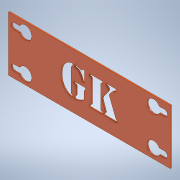
# Autodesk Inventor part: Head_GK_cloth
Saved by Autodesk Inventor 2020.4 (Build 244396000, 396)
## iProperties
Created: 2022-06-21
Part Number: Head_GK_cloth
Material: 一般
Document SubType Name: Modeling
Designer: Masato Kubotera
Density: 1 g/cm^3
Appearance: 滑らか - 淡いオレンジ
Author: Masato Kubotera
Autodesk Inventor part; units mm, degrees
ref_plane "YZ Plane" through (0, 0, 0) normal (1, 0, 0) x (0, 1, 0)
ref_plane "XZ Plane" through (0, 0, 0) normal (0, 1, 0) x (-1, 0, 0)
ref_plane "XY Plane" through (0, 0, 0) normal (0, 0, 1) x (1, 0, 0)
sketch "スケッチ1" plane through (0, 0, 0) normal (1, 0, 0) x (0, 1, 0)
  line L0 (-56.1, 19) -> (56.1, 19)
  line L1 (56.1, 19) -> (56.1, -19)
  line L2 (56.1, -19) -> (-56.1, -19)
  line L3 (-56.1, -19) -> (-56.1, 19)
  line L4 (-56.1, 19) -> (56.1, -19) construction
  line L5 (56.1, 19) -> (-56.1, -19) construction
  arc A0 (-48.4799, 10.4) -> (-48.4799, 14.6) centre (-44.5, 12.5) ccw
  line L6 (-52, 10.4) -> (-48.4799, 10.4)
  line L7 (-52, 14.6) -> (-48.4799, 14.6)
  arc A1 (-52, 14.6) -> (-52, 10.4) centre (-52, 12.5) ccw
  line L8 (-52, 12.5) -> (-44.5, 12.5) construction
  line L9 (-56.1, 0) -> (56.1, 0) construction
  line L10 (-52, 19) -> (-52, -19) construction
  line L11 (-56.1, -19) -> (56.1, 19) construction
  line L12 (-52, -14.6) -> (-48.4799, -14.6)
  arc A2 (-52, -10.4) -> (-52, -14.6) centre (-52, -12.5) ccw
  line L13 (-52, -10.4) -> (-48.4799, -10.4)
  arc A3 (-48.4799, -14.6) -> (-48.4799, -10.4) centre (-44.5, -12.5) ccw
  line L14 (-52, -12.5) -> (-44.5, -12.5) construction
  line L15 (-52, -19) -> (-52, 19) construction
  line L16 (0, 19) -> (0, -19) construction
  line L17 (56.1, 19) -> (-56.1, -19) construction
  line L18 (-56.1, 19) -> (56.1, -19) construction
  line L19 (52, 14.6) -> (48.4799, 14.6)
  arc A4 (52, 10.4) -> (52, 14.6) centre (52, 12.5) ccw
  line L20 (52, 10.4) -> (48.4799, 10.4)
  arc A5 (48.4799, 14.6) -> (48.4799, 10.4) centre (44.5, 12.5) ccw
  line L21 (52, 12.5) -> (44.5, 12.5) construction
  line L22 (56.1, 0) -> (-56.1, 0) construction
  line L23 (52, 19) -> (52, -19) construction
  arc A6 (52, -14.6) -> (52, -10.4) centre (52, -12.5) ccw
  line L24 (52, -14.6) -> (48.4799, -14.6)
  line L25 (52, -10.4) -> (48.4799, -10.4)
  line L26 (52, -12.5) -> (44.5, -12.5) construction
  arc A7 (48.4799, -10.4) -> (48.4799, -14.6) centre (44.5, -12.5) ccw
  line L27 (52, -19) -> (52, 19) construction
  line L28 (56.1, -19) -> (-56.1, 19) construction
  line L29 (-9.8507, 5.0432) -> (9.8507, 5.0432) construction
  line L30 (9.8507, 5.0432) -> (9.8507, -5.0432) construction
  line L31 (9.8507, -5.0432) -> (-9.8507, -5.0432) construction
  line L32 (-9.8507, -5.0432) -> (-9.8507, 5.0432) construction
  line L33 (-9.8507, 5.0432) -> (9.8507, -5.0432) construction
  line L34 (9.8507, 5.0432) -> (-9.8507, -5.0432) construction
  line L35 (-11.4757, 10.3993) -> (-11.4757, 8.7674)
  spline S0 degree 2 poles (-11.4757, 8.7674) (-12.7604, 8.4549) (-12.7604, 6.7187) knots 0 0 0 1 1 1
  line L36 (-12.7604, 6.7187) -> (-12.7604, -6.9271)
  spline S1 degree 2 poles (-12.7604, -6.9271) (-12.7604, -7.7083) (-12.5347, -8.1424) knots 0 0 0 1 1 1
  spline S2 degree 2 poles (-12.5347, -8.1424) (-12.3437, -8.4896) (-11.7361, -8.7326) knots 0 0 0 1 1 1
  line L37 (-11.7361, -8.7326) -> (-11.7361, -10.3993)
  spline S3 degree 2 poles (-11.7361, -10.3993) (-12.2049, -10.3993) (-12.9861, -10.2431) (-13.6285, -10.0347) knots 0 0 0 1 2 2 2
  spline S4 degree 2 poles (-13.6285, -10.0347) (-15.1562, -9.4965) (-17.6562, -7.3264) (-18.4549, -5.816) knots 0 0 0 1 2 2 2
  spline S5 degree 2 poles (-18.4549, -5.816) (-19.7049, -3.4722) (-19.7049, -0.2431) knots 0 0 0 1 1 1
  spline S6 degree 2 poles (-19.7049, -0.2431) (-19.7049, 2.8819) (-17.4826, 7.7083) (-15.3993, 9.0972) knots 0 0 0 1 2 2 2
  spline S7 degree 2 poles (-15.3993, 9.0972) (-14.2014, 9.8958) (-12.8299, 10.2431) knots 0 0 0 1 1 1
  spline S8 degree 2 poles (-12.8299, 10.2431) (-12.2569, 10.3993) (-11.4757, 10.3993) knots 0 0 0 1 1 1
  spline S9 degree 2 poles (-3.6632, -7.5521) (-4.2535, -8.1424) (-6.1979, -9.3576) (-7.066, -9.7049) knots 0 0 0 1 2 2 2
  spline S10 degree 2 poles (-7.066, -9.7049) (-7.8472, -10.0174) (-9.7743, -10.3993) (-10.5035, -10.3993) knots 0 0 0 1 2 2 2
  line L38 (-10.5035, -10.3993) -> (-10.5035, -8.7326)
  spline S11 degree 2 poles (-10.5035, -8.7326) (-10.0694, -8.6458) (-9.6528, -8.3507) (-9.4965, -8.0729) knots 0 0 0 1 2 2 2
  spline S12 degree 2 poles (-9.4965, -8.0729) (-9.2535, -7.6215) (-9.2535, -6.9271) knots 0 0 0 1 1 1
  line L39 (-9.2535, -6.9271) -> (-9.2535, -2.6389)
  spline S13 degree 2 poles (-9.2535, -2.6389) (-9.2535, -2.066) (-9.4792, -1.8229) knots 0 0 0 1 1 1
  spline S14 degree 2 poles (-9.4792, -1.8229) (-9.5833, -1.684) (-9.7743, -1.5972) (-10.3472, -1.4757) knots 0 0 0 1 2 2 2
  spline S15 degree 2 poles (-10.3472, -1.4757) (-11.059, -1.3021) (-11.059, -0.6597) knots 0 0 0 1 1 1
  spline S16 degree 2 poles (-11.059, -0.6597) (-11.059, -0.2778) (-10.3993, 0.1389) (-9.7569, 0.1389) knots 0 0 0 1 2 2 2
  line L40 (-9.7569, 0.1389) -> (-9.2708, 0.1389)
  line L41 (-9.2708, 0.1389) -> (-3.9062, 0.1389)
  spline S17 degree 2 poles (-3.9062, 0.1389) (-3.2465, 0.1389) (-2.7083, -0.2257) (-2.7083, -0.6771) knots 0 0 0 1 2 2 2
  spline S18 degree 2 poles (-2.7083, -0.6771) (-2.7083, -0.9549) (-2.934, -1.3194) (-3.2292, -1.5278) knots 0 0 0 1 2 2 2
  spline S19 degree 2 poles (-3.2292, -1.5278) (-3.5243, -1.7361) (-3.6632, -2.0833) (-3.6632, -2.5521) knots 0 0 0 1 2 2 2
  line L42 (-3.6632, -2.5521) -> (-3.6632, -7.5521)
  line L43 (-10.2778, 8.8021) -> (-10.2778, 10.3819)
  spline S20 degree 2 poles (-10.2778, 10.3819) (-7.8993, 10.1562) (-6.3542, 9.4965) knots 0 0 0 1 1 1
  spline S21 degree 2 poles (-6.3542, 9.4965) (-5.9028, 9.2882) (-5.6597, 9.2882) knots 0 0 0 1 1 1
  spline S22 degree 2 poles (-5.6597, 9.2882) (-5.4167, 9.2882) (-5.1736, 9.5139) (-4.7917, 10.0347) knots 0 0 0 1 2 2 2
  spline S23 degree 2 poles (-4.7917, 10.0347) (-4.5312, 10.3993) (-4.1319, 10.3993) knots 0 0 0 1 1 1
  spline S24 degree 2 poles (-4.1319, 10.3993) (-3.7153, 10.3993) (-3.3854, 9.9479) (-3.3854, 9.4097) knots 0 0 0 1 2 2 2
  line L44 (-3.3854, 9.4097) -> (-3.3854, 3.7153)
  spline S25 degree 2 poles (-3.3854, 3.7153) (-3.3854, 2.5868) (-4.2014, 2.5868) knots 0 0 0 1 1 1
  spline S26 degree 2 poles (-4.2014, 2.5868) (-4.6181, 2.5868) (-5.0174, 3.0208) (-5.191, 3.6806) knots 0 0 0 1 2 2 2
  spline S27 degree 2 poles (-5.191, 3.6806) (-5.3993, 4.4965) (-6.5451, 6.684) (-7.066, 7.309) knots 0 0 0 1 2 2 2
  spline S28 degree 2 poles (-7.066, 7.309) (-7.6736, 8.0556) (-9.1667, 8.7326) (-10.2778, 8.8021) knots 0 0 0 1 2 2 2
  line L45 (7.8299, -10) -> (1.2847, -10)
  line L46 (1.2847, -10) -> (0.9028, -10)
  spline S29 degree 2 poles (0.9028, -10) (0.3819, -10) (-0.191, -9.6007) (-0.191, -9.2361) knots 0 0 0 1 2 2 2
  spline S30 degree 2 poles (-0.191, -9.2361) (-0.191, -8.6458) (0.3993, -8.4549) knots 0 0 0 1 1 1
  spline S31 degree 2 poles (0.3993, -8.4549) (0.8854, -8.2813) (1.0417, -8.2118) (1.1285, -8.0729) knots 0 0 0 1 2 2 2
  spline S32 degree 2 poles (1.1285, -8.0729) (1.3021, -7.8472) (1.3021, -7.3264) knots 0 0 0 1 1 1
  line L47 (1.3021, -7.3264) -> (1.3021, 7.3264)
  spline S33 degree 2 poles (1.3021, 7.3264) (1.3021, 7.8472) (1.1285, 8.0729) knots 0 0 0 1 1 1
  spline S34 degree 2 poles (1.1285, 8.0729) (1.0417, 8.2118) (0.8854, 8.2812) (0.3993, 8.4375) knots 0 0 0 1 2 2 2
  spline S35 degree 2 poles (0.3993, 8.4375) (-0.191, 8.6285) (-0.191, 9.2361) knots 0 0 0 1 1 1
  spline S36 degree 2 poles (-0.191, 9.2361) (-0.191, 9.6007) (0.3819, 10) (0.9028, 10) knots 0 0 0 1 2 2 2
  line L48 (0.9028, 10) -> (1.2847, 10)
  line L49 (1.2847, 10) -> (7.8299, 10)
  line L50 (7.8299, 10) -> (8.2118, 10)
  spline S37 degree 2 poles (8.2118, 10) (8.7326, 10) (9.3056, 9.6007) (9.3056, 9.2361) knots 0 0 0 1 2 2 2
  spline S38 degree 2 poles (9.3056, 9.2361) (9.3056, 8.6285) (8.7153, 8.4375) knots 0 0 0 1 1 1
  spline S39 degree 2 poles (8.7153, 8.4375) (8.2292, 8.2812) (8.0729, 8.2118) (7.9861, 8.0729) knots 0 0 0 1 2 2 2
  spline S40 degree 2 poles (7.9861, 8.0729) (7.8125, 7.8472) (7.8125, 7.3264) knots 0 0 0 1 1 1
  line L51 (7.8125, 7.3264) -> (7.8125, -7.3264)
  spline S41 degree 2 poles (7.8125, -7.3264) (7.8125, -8.1597) (8.2465, -8.2986) knots 0 0 0 1 1 1
  line L52 (8.2465, -8.2986) -> (8.6979, -8.4549)
  spline S42 degree 2 poles (8.6979, -8.4549) (9.2535, -8.6285) (9.2535, -9.2361) knots 0 0 0 1 1 1
  spline S43 degree 2 poles (9.2535, -9.2361) (9.2535, -10) (8.2118, -10) knots 0 0 0 1 1 1
  line L53 (8.2118, -10) -> (7.8299, -10)
  line L54 (13.6285, 4.184) -> (18.0556, -7.3785)
  spline S44 degree 2 poles (18.0556, -7.3785) (18.2292, -7.8472) (18.6111, -8.3333) (18.9062, -8.4549) knots 0 0 0 1 2 2 2
  spline S45 degree 2 poles (18.9062, -8.4549) (19.2188, -8.6111) (19.3056, -8.6806) knots 0 0 0 1 1 1
  spline S46 degree 2 poles (19.3056, -8.6806) (19.5139, -8.8889) (19.5139, -9.2188) knots 0 0 0 1 1 1
  spline S47 degree 2 poles (19.5139, -9.2188) (19.5139, -10) (18.4028, -10) knots 0 0 0 1 1 1
  line L55 (18.4028, -10) -> (11.0417, -10)
  spline S48 degree 2 poles (11.0417, -10) (10.5208, -10) (9.9479, -9.566) (9.9479, -9.1493) knots 0 0 0 1 2 2 2
  spline S49 degree 2 poles (9.9479, -9.1493) (9.9479, -8.6806) (10.4861, -8.4201) knots 0 0 0 1 1 1
  spline S50 degree 2 poles (10.4861, -8.4201) (10.8333, -8.2639) (11.059, -8.0382) (11.0764, -7.8472) knots 0 0 0 1 2 2 2
  spline S51 degree 2 poles (11.0764, -7.8472) (11.0764, -7.7431) (10.9549, -7.3785) knots 0 0 0 1 1 1
  line L56 (10.9549, -7.3785) -> (9.0799, -1.7882)
  spline S52 degree 2 poles (9.0799, -1.7882) (8.8194, -1.0069) (8.8194, -0.4688) knots 0 0 0 1 1 1
  spline S53 degree 2 poles (8.8194, -0.4688) (8.8194, 0.0521) (9.2361, 0.6597) knots 0 0 0 1 1 1
  line L57 (9.2361, 0.6597) -> (12.7431, 5.5903)
  spline S54 degree 2 poles (12.7431, 5.5903) (13.2465, 6.2847) (13.2465, 7.0312) knots 0 0 0 1 1 1
  spline S55 degree 2 poles (13.2465, 7.0312) (13.2465, 7.4306) (12.8125, 8.1424) (12.4306, 8.2812) knots 0 0 0 1 2 2 2
  line L58 (12.4306, 8.2812) -> (11.9097, 8.5069)
  spline S56 degree 2 poles (11.9097, 8.5069) (11.4063, 8.7153) (11.4063, 9.2014) knots 0 0 0 1 1 1
  spline S57 degree 2 poles (11.4063, 9.2014) (11.4063, 9.5833) (11.7188, 9.8437) knots 0 0 0 1 1 1
  spline S58 degree 2 poles (11.7188, 9.8437) (11.9271, 10) (12.3958, 10) knots 0 0 0 1 1 1
  line L59 (12.3958, 10) -> (17.6042, 10)
  spline S59 degree 2 poles (17.6042, 10) (18.125, 10) (18.6979, 9.5486) (18.6979, 9.1319) knots 0 0 0 1 2 2 2
  spline S60 degree 2 poles (18.6979, 9.1319) (18.6979, 8.5243) (18.0208, 8.2465) knots 0 0 0 1 1 1
  line L60 (18.0208, 8.2465) -> (17.2396, 7.9514)
  spline S61 degree 2 poles (17.2396, 7.9514) (16.7535, 7.7778) (16.0069, 7.1528) knots 0 0 0 1 1 1
  spline S62 degree 2 poles (16.0069, 7.1528) (15.4514, 6.684) (14.6354, 5.5903) knots 0 0 0 1 1 1
  line L61 (14.6354, 5.5903) -> (13.6285, 4.184)
  line L62 (-11.4757, 10.3993) -> (-11.4757, 8.7674)
  spline S63 degree 2 poles (-11.4757, 8.7674) (-12.7604, 8.4549) (-12.7604, 6.7187) knots 0 0 0 1 1 1
  line L63 (-12.7604, 6.7187) -> (-12.7604, -6.9271)
  spline S64 degree 2 poles (-12.7604, -6.9271) (-12.7604, -7.7083) (-12.5347, -8.1424) knots 0 0 0 1 1 1
  spline S65 degree 2 poles (-12.5347, -8.1424) (-12.3437, -8.4896) (-11.7361, -8.7326) knots 0 0 0 1 1 1
  line L64 (-11.7361, -8.7326) -> (-11.7361, -10.3993)
  spline S66 degree 2 poles (-11.7361, -10.3993) (-12.2049, -10.3993) (-12.9861, -10.2431) (-13.6285, -10.0347) knots 0 0 0 1 2 2 2
  spline S67 degree 2 poles (-13.6285, -10.0347) (-15.1562, -9.4965) (-17.6562, -7.3264) (-18.4549, -5.816) knots 0 0 0 1 2 2 2
  spline S68 degree 2 poles (-18.4549, -5.816) (-19.7049, -3.4722) (-19.7049, -0.2431) knots 0 0 0 1 1 1
  spline S69 degree 2 poles (-19.7049, -0.2431) (-19.7049, 2.8819) (-17.4826, 7.7083) (-15.3993, 9.0972) knots 0 0 0 1 2 2 2
  spline S70 degree 2 poles (-15.3993, 9.0972) (-14.2014, 9.8958) (-12.8299, 10.2431) knots 0 0 0 1 1 1
  spline S71 degree 2 poles (-12.8299, 10.2431) (-12.2569, 10.3993) (-11.4757, 10.3993) knots 0 0 0 1 1 1
  spline S72 degree 2 poles (-3.6632, -7.5521) (-4.2535, -8.1424) (-6.1979, -9.3576) (-7.066, -9.7049) knots 0 0 0 1 2 2 2
  spline S73 degree 2 poles (-7.066, -9.7049) (-7.8472, -10.0174) (-9.7743, -10.3993) (-10.5035, -10.3993) knots 0 0 0 1 2 2 2
  line L65 (-10.5035, -10.3993) -> (-10.5035, -8.7326)
  spline S74 degree 2 poles (-10.5035, -8.7326) (-10.0694, -8.6458) (-9.6528, -8.3507) (-9.4965, -8.0729) knots 0 0 0 1 2 2 2
  spline S75 degree 2 poles (-9.4965, -8.0729) (-9.2535, -7.6215) (-9.2535, -6.9271) knots 0 0 0 1 1 1
  line L66 (-9.2535, -6.9271) -> (-9.2535, -2.6389)
  spline S76 degree 2 poles (-9.2535, -2.6389) (-9.2535, -2.066) (-9.4792, -1.8229) knots 0 0 0 1 1 1
  spline S77 degree 2 poles (-9.4792, -1.8229) (-9.5833, -1.684) (-9.7743, -1.5972) (-10.3472, -1.4757) knots 0 0 0 1 2 2 2
  spline S78 degree 2 poles (-10.3472, -1.4757) (-11.059, -1.3021) (-11.059, -0.6597) knots 0 0 0 1 1 1
  spline S79 degree 2 poles (-11.059, -0.6597) (-11.059, -0.2778) (-10.3993, 0.1389) (-9.7569, 0.1389) knots 0 0 0 1 2 2 2
  line L67 (-9.7569, 0.1389) -> (-9.2708, 0.1389)
  line L68 (-9.2708, 0.1389) -> (-3.9062, 0.1389)
  spline S80 degree 2 poles (-3.9062, 0.1389) (-3.2465, 0.1389) (-2.7083, -0.2257) (-2.7083, -0.6771) knots 0 0 0 1 2 2 2
  spline S81 degree 2 poles (-2.7083, -0.6771) (-2.7083, -0.9549) (-2.934, -1.3194) (-3.2292, -1.5278) knots 0 0 0 1 2 2 2
  spline S82 degree 2 poles (-3.2292, -1.5278) (-3.5243, -1.7361) (-3.6632, -2.0833) (-3.6632, -2.5521) knots 0 0 0 1 2 2 2
  line L69 (-3.6632, -2.5521) -> (-3.6632, -7.5521)
  line L70 (-10.2778, 8.8021) -> (-10.2778, 10.3819)
  spline S83 degree 2 poles (-10.2778, 10.3819) (-7.8993, 10.1562) (-6.3542, 9.4965) knots 0 0 0 1 1 1
  spline S84 degree 2 poles (-6.3542, 9.4965) (-5.9028, 9.2882) (-5.6597, 9.2882) knots 0 0 0 1 1 1
  spline S85 degree 2 poles (-5.6597, 9.2882) (-5.4167, 9.2882) (-5.1736, 9.5139) (-4.7917, 10.0347) knots 0 0 0 1 2 2 2
  spline S86 degree 2 poles (-4.7917, 10.0347) (-4.5312, 10.3993) (-4.1319, 10.3993) knots 0 0 0 1 1 1
  spline S87 degree 2 poles (-4.1319, 10.3993) (-3.7153, 10.3993) (-3.3854, 9.9479) (-3.3854, 9.4097) knots 0 0 0 1 2 2 2
  line L71 (-3.3854, 9.4097) -> (-3.3854, 3.7153)
  spline S88 degree 2 poles (-3.3854, 3.7153) (-3.3854, 2.5868) (-4.2014, 2.5868) knots 0 0 0 1 1 1
  spline S89 degree 2 poles (-4.2014, 2.5868) (-4.6181, 2.5868) (-5.0174, 3.0208) (-5.191, 3.6806) knots 0 0 0 1 2 2 2
  spline S90 degree 2 poles (-5.191, 3.6806) (-5.3993, 4.4965) (-6.5451, 6.684) (-7.066, 7.309) knots 0 0 0 1 2 2 2
  spline S91 degree 2 poles (-7.066, 7.309) (-7.6736, 8.0556) (-9.1667, 8.7326) (-10.2778, 8.8021) knots 0 0 0 1 2 2 2
  line L72 (7.8299, -10) -> (1.2847, -10)
  line L73 (1.2847, -10) -> (0.9028, -10)
  spline S92 degree 2 poles (0.9028, -10) (0.3819, -10) (-0.191, -9.6007) (-0.191, -9.2361) knots 0 0 0 1 2 2 2
  spline S93 degree 2 poles (-0.191, -9.2361) (-0.191, -8.6458) (0.3993, -8.4549) knots 0 0 0 1 1 1
  spline S94 degree 2 poles (0.3993, -8.4549) (0.8854, -8.2813) (1.0417, -8.2118) (1.1285, -8.0729) knots 0 0 0 1 2 2 2
  spline S95 degree 2 poles (1.1285, -8.0729) (1.3021, -7.8472) (1.3021, -7.3264) knots 0 0 0 1 1 1
  line L74 (1.3021, -7.3264) -> (1.3021, 7.3264)
  spline S96 degree 2 poles (1.3021, 7.3264) (1.3021, 7.8472) (1.1285, 8.0729) knots 0 0 0 1 1 1
  spline S97 degree 2 poles (1.1285, 8.0729) (1.0417, 8.2118) (0.8854, 8.2812) (0.3993, 8.4375) knots 0 0 0 1 2 2 2
  spline S98 degree 2 poles (0.3993, 8.4375) (-0.191, 8.6285) (-0.191, 9.2361) knots 0 0 0 1 1 1
  spline S99 degree 2 poles (-0.191, 9.2361) (-0.191, 9.6007) (0.3819, 10) (0.9028, 10) knots 0 0 0 1 2 2 2
  line L75 (0.9028, 10) -> (1.2847, 10)
  line L76 (1.2847, 10) -> (7.8299, 10)
  line L77 (7.8299, 10) -> (8.2118, 10)
  spline S100 degree 2 poles (8.2118, 10) (8.7326, 10) (9.3056, 9.6007) (9.3056, 9.2361) knots 0 0 0 1 2 2 2
  spline S101 degree 2 poles (9.3056, 9.2361) (9.3056, 8.6285) (8.7153, 8.4375) knots 0 0 0 1 1 1
  spline S102 degree 2 poles (8.7153, 8.4375) (8.2292, 8.2812) (8.0729, 8.2118) (7.9861, 8.0729) knots 0 0 0 1 2 2 2
  spline S103 degree 2 poles (7.9861, 8.0729) (7.8125, 7.8472) (7.8125, 7.3264) knots 0 0 0 1 1 1
  line L78 (7.8125, 7.3264) -> (7.8125, -7.3264)
  spline S104 degree 2 poles (7.8125, -7.3264) (7.8125, -8.1597) (8.2465, -8.2986) knots 0 0 0 1 1 1
  line L79 (8.2465, -8.2986) -> (8.6979, -8.4549)
  spline S105 degree 2 poles (8.6979, -8.4549) (9.2535, -8.6285) (9.2535, -9.2361) knots 0 0 0 1 1 1
  spline S106 degree 2 poles (9.2535, -9.2361) (9.2535, -10) (8.2118, -10) knots 0 0 0 1 1 1
  line L80 (8.2118, -10) -> (7.8299, -10)
  line L81 (13.6285, 4.184) -> (18.0556, -7.3785)
  spline S107 degree 2 poles (18.0556, -7.3785) (18.2292, -7.8472) (18.6111, -8.3333) (18.9062, -8.4549) knots 0 0 0 1 2 2 2
  spline S108 degree 2 poles (18.9062, -8.4549) (19.2188, -8.6111) (19.3056, -8.6806) knots 0 0 0 1 1 1
  spline S109 degree 2 poles (19.3056, -8.6806) (19.5139, -8.8889) (19.5139, -9.2188) knots 0 0 0 1 1 1
  spline S110 degree 2 poles (19.5139, -9.2188) (19.5139, -10) (18.4028, -10) knots 0 0 0 1 1 1
  line L82 (18.4028, -10) -> (11.0417, -10)
  spline S111 degree 2 poles (11.0417, -10) (10.5208, -10) (9.9479, -9.566) (9.9479, -9.1493) knots 0 0 0 1 2 2 2
  spline S112 degree 2 poles (9.9479, -9.1493) (9.9479, -8.6806) (10.4861, -8.4201) knots 0 0 0 1 1 1
  spline S113 degree 2 poles (10.4861, -8.4201) (10.8333, -8.2639) (11.059, -8.0382) (11.0764, -7.8472) knots 0 0 0 1 2 2 2
  spline S114 degree 2 poles (11.0764, -7.8472) (11.0764, -7.7431) (10.9549, -7.3785) knots 0 0 0 1 1 1
  line L83 (10.9549, -7.3785) -> (9.0799, -1.7882)
  spline S115 degree 2 poles (9.0799, -1.7882) (8.8194, -1.0069) (8.8194, -0.4688) knots 0 0 0 1 1 1
  spline S116 degree 2 poles (8.8194, -0.4688) (8.8194, 0.0521) (9.2361, 0.6597) knots 0 0 0 1 1 1
  line L84 (9.2361, 0.6597) -> (12.7431, 5.5903)
  spline S117 degree 2 poles (12.7431, 5.5903) (13.2465, 6.2847) (13.2465, 7.0312) knots 0 0 0 1 1 1
  spline S118 degree 2 poles (13.2465, 7.0312) (13.2465, 7.4306) (12.8125, 8.1424) (12.4306, 8.2812) knots 0 0 0 1 2 2 2
  line L85 (12.4306, 8.2812) -> (11.9097, 8.5069)
  spline S119 degree 2 poles (11.9097, 8.5069) (11.4063, 8.7153) (11.4063, 9.2014) knots 0 0 0 1 1 1
  spline S120 degree 2 poles (11.4063, 9.2014) (11.4063, 9.5833) (11.7188, 9.8437) knots 0 0 0 1 1 1
  spline S121 degree 2 poles (11.7188, 9.8437) (11.9271, 10) (12.3958, 10) knots 0 0 0 1 1 1
  line L86 (12.3958, 10) -> (17.6042, 10)
  spline S122 degree 2 poles (17.6042, 10) (18.125, 10) (18.6979, 9.5486) (18.6979, 9.1319) knots 0 0 0 1 2 2 2
  spline S123 degree 2 poles (18.6979, 9.1319) (18.6979, 8.5243) (18.0208, 8.2465) knots 0 0 0 1 1 1
  line L87 (18.0208, 8.2465) -> (17.2396, 7.9514)
  spline S124 degree 2 poles (17.2396, 7.9514) (16.7535, 7.7778) (16.0069, 7.1528) knots 0 0 0 1 1 1
  spline S125 degree 2 poles (16.0069, 7.1528) (15.4514, 6.684) (14.6354, 5.5903) knots 0 0 0 1 1 1
  line L88 (14.6354, 5.5903) -> (13.6285, 4.184)
  point P0 (0, 0)
  point P1 (0, 5.0432)
  point P2 (0, 0)
  dimension "d0" = 112.2
  dimension "d1" = 9
  dimension "d2" = 4.2
  dimension "d3" = 7.5
  dimension "d5" = 2
  dimension "d6" = 25
  dimension "d7" = 2
  dimension "d8" = 38
  constraints: 62 end point, 30 symmetric about line, 16 point on circle, 9 midpoint, 8 centre point, 7 point on line, 4 parallel, 2 perpendicular, 2 tangent, 1 horizontal, 9 other
  measures "d0" distance of L1.end L2.end
  measures "d1" diameter of A0
  measures "d2" diameter of A1
  measures "d3" distance of L8.start L8.end
  measures "d5" distance edge to line of A1 L3
  measures "d6" distance of L14.start L8.start
  measures "d7" distance edge to line of A0 L0
  measures "d8" distance of L0.end L1.end
extrude "押し出し1" add sketch "スケッチ1" along normal blind 0.75 contours L0 L1 L2 L3 | L35 S0 L36 S1 S2 L37 S3 S4 S5 S6 S7 S8 | S9 S10 L38 S11 S12 L39 S13 S14 S15 S16 L40 L41 S17 S18 S19 L42 | L43 S20 S21 S22 S23 S24 L44 S25 S26 S27 S28 | L45 L46 S29 S30 S31 S32 L47 S33 S34 S35 S36 L48 L49 L50 S37 S38 S39 S40 L51 S41 L52 S42 S43 L53 | L54 S44 S45 S46 S47 L55 S48 S49 S50 S51 L56 S52 S53 L57 S54 S55 L58 S56 S57 S58 L59 S59 S60 L60 S61 S62 L61
extrude "押し出し2" cut sketch "スケッチ1" along normal through all contours L35 S0 L36 S1 S2 L37 S3 S4 S5 S6 S7 S8 | S9 S10 L38 S11 S12 L39 S13 S14 S15 S16 L40 L41 S17 S18 S19 L42 | L43 S20 S21 S22 S23 S24 L44 S25 S26 S27 S28 | L45 L46 S29 S30 S31 S32 L47 S33 S34 S35 S36 L48 L49 L50 S37 S38 S39 S40 L51 S41 L52 S42 S43 L53 | L54 S44 S45 S46 S47 L55 S48 S49 S50 S51 L56 S52 S53 L57 S54 S55 L58 S56 S57 S58 L59 S59 S60 L60 S61 S62 L61
equation "\"d7\" = d5"
